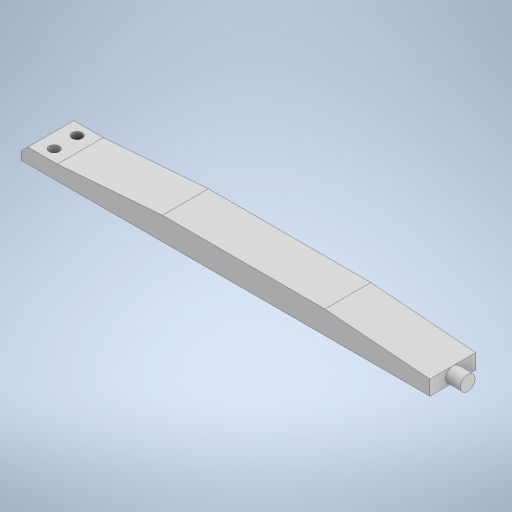
# Autodesk Inventor part: pieza 1-29
Saved by Autodesk Inventor 2024.2 (Build 282272000, 272)
## iProperties
Created: 2024-10-10
Part Number: pieza 1-29
Material: Generic
Document SubType Name: Modeling
Designer: Precisión-18
Density: 1 g/cm^3
Appearance: Default
Author: Precisión-18
Autodesk Inventor part; units mm, degrees
ref_plane "YZ Plane" through (0, 0, 0) normal (1, 0, 0) x (0, 1, 0)
ref_plane "XZ Plane" through (0, 0, 0) normal (0, 1, 0) x (-1, 0, 0)
ref_plane "XY Plane" through (0, 0, 0) normal (0, 0, 1) x (1, 0, 0)
sketch "Sketch1" plane through (0, 0, 0) normal (0, 0, 1) x (1, 0, 0)
  line L0 (0, 0) -> (0, 2.5)
  line L1 (2, 4.5) -> (11, 4.5)
  line L2 (0, 2.5) -> (2, 4.5)
  line L3 (0, 8.8411) -> (0, 0) construction
  line L4 (43, 7) -> (92.5, 7)
  line L5 (43, 11.0001) -> (43, -2.4525) construction
  line L6 (43, 7) -> (11, 4.5)
  line L7 (92.5, 7) -> (124.5, 4.5)
  line L8 (0, 0) -> (149.0621, 0)
  line L9 (124.5, 4.5) -> (124.5, 0)
  dimension "d0" = 4.5
  dimension "d1" = 45
  dimension "d2" = 7
  dimension "d3" = 9
  dimension "d4" = 32
  dimension "d5" = 49.5
  dimension "d8" = 32
  dimension "d9" = 2
  dimension "d10" = 4.5
  constraints: 20 end point, 3 horizontal, 3 vertical, 2 point on line, 1 perpendicular
  measures "d0" distance from line of L0.start L1
  measures "d1" angle of L3 L2
  measures "d2" distance from line of L0.start L4
  measures "d3" distance of L1.start L1.end
  measures "d4" distance from line of L5 L1.end
  measures "d5" distance of L4.end L4.start
  measures "d8" horizontal distance of L7.end L4.end
  measures "d9" horizontal distance of L0.end L1.start
  measures "d10" distance of L7.end L9.end
extrude "Extrusion1" add sketch "Sketch1" along normal blind 14
sketch "Sketch2" plane through (124.5, 0, 0) normal (1, 0, 0) x (0, 0, -1)
  circle A0 centre (-7, 2.25) radius 2.25
  line L0 (0, 4.5) -> (-14, 4.5) projected
  line L1 (-7, 4.5) -> (-7, -0.9771) construction
  line L2 (0, 2.5) -> (-14, 2.5) projected
  point P0 (0, 0)
  dimension "d13" = 4.5
  constraints: 2 end point, 1 centre point, 1 midpoint, 1 perpendicular, 1 point on line, 1 tangent
  measures "d13" diameter of A0
extrude "Extrusion2" add sketch "Sketch2" along normal blind 4.5
sketch "Sketch3" plane through (2, 4.5, 0) normal (0, 1, 0) x (1, 0, 0)
  circle A0 centre (4.5, -3.5) radius 1.5
  circle A1 centre (4.5, -10.5) radius 1.5
  line L0 (9, 0) -> (0, 0) projected
  line L1 (9, -14) -> (0, -14) projected
  line L2 (0, 0) -> (0, -14) projected
  point P0 (-2, 0)
  dimension "d16" = 7
  dimension "d17" = 3.5
  dimension "d18" = 3.5
  dimension "d19" = 4.5
  dimension "d20" = 3
  dimension "d21" = 3
  constraints: 2 centre point
  measures "d16" distance of A1.centre A0.centre
  measures "d17" distance from line of L0 A0.centre
  measures "d18" distance from line of L1 A1.centre
  measures "d19" distance from line of L2 A1.centre
  measures "d20" diameter of A0
  measures "d21" diameter of A1
extrude "Extrusion3" cut sketch "Sketch3" against normal blind 4.5
body "Solid1"
